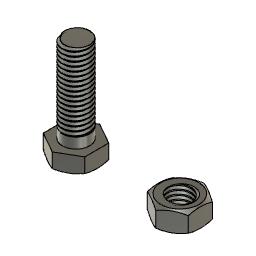
screw v1 (Autodesk Fusion 360 design; units mm, degrees)
Autodesk Fusion 360 part; units mm, degrees
sketch "Sketch1" plane through (0, 0, 0) normal (0, 0, 1) x (1, 0, 0)
  line L0 (6.0104, -3.446) -> (5.9895, 3.4822)
  line L1 (5.9895, 3.4822) -> (-0.0209, 6.9282)
  line L2 (-0.0209, 6.9282) -> (-6.0104, 3.446)
  line L3 (-6.0104, 3.446) -> (-5.9895, -3.4822)
  line L4 (-5.9895, -3.4822) -> (0.0209, -6.9282)
  line L5 (0.0209, -6.9282) -> (6.0104, -3.446)
  circle A0 centre (0, 0) radius 5.5
  circle A1 centre (0, 0) radius 4
  dimension "d1" = 6
  dimension "d2" = 11
  dimension "d3" = 8
  constraint coincident A0.centre A1.centre
  measures "d1" distance of A0.centre L5
  measures "d2" diameter of A0
  measures "d3" diameter of A1
extrude "Extrude1" add sketch "Sketch1" along normal blind 5 contours L0 L1 L2 L3 L4 L5 | A0 | A1 makes body 1
extrude "Extrude2" cut sketch "Sketch1" along normal blind 12.535 draft 60 contours A0 keep common part bodies 1
extrude "Extrude3" add sketch "Sketch1" along normal blind 30 contours A1 bodies 1
thread "Thread1" "ISO Metric profile 8.0 M8x1.25 6g" major diameter 7.866 minor diameter 6.4455 pitch 1.25 angle 60 modelled right hand crest width 0.1833 on face at (3.9801, 0.3983, 13.3333) from (0, 0, 8) to (0, 0, 30) crest through (3.933, 0, 4.6875) on bodies 1
sketch "Sketch2" plane through (0, 0, 0) normal (0, 0, 1) x (1, 0, 0)
  line L0 (35.9472, -3.4041) -> (36.0159, 3.5237)
  line L1 (36.0159, 3.5237) -> (30.0505, 7.0471)
  line L2 (30.0505, 7.0471) -> (24.0164, 3.6427)
  line L3 (24.0164, 3.6427) -> (23.9478, -3.2852)
  line L4 (23.9478, -3.2852) -> (29.9132, -6.8086)
  line L5 (29.9132, -6.8086) -> (35.9472, -3.4041)
  circle A0 centre (29.9818, 0.1193) radius 5.5
  circle A1 centre (29.9818, 0.1193) radius 4
  point P0 (29.9818, 0.1193)
  dimension "d12" = 6
  dimension "d13" = 11
  dimension "d14" = 8
  constraint coincident P0 A0.centre
  constraint concentric A0 A1
  measures "d12" distance of P0 L5
  measures "d13" diameter of A0
  measures "d14" diameter of A1
extrude "Extrude4" add sketch "Sketch2" along normal blind 6 separate body contours L0 L1 L2 L3 L4 L5 | A0 makes body 2
sketch "Sketch3" plane through (0, 0, 0) normal (0, 0, 1) x (1, 0, 0)
  circle A0 centre (29.976, -0.0398) radius 5.5
  dimension "d17" = 11
  measures "d17" diameter of A0
extrude "Extrude5" cut sketch "Sketch3" along normal blind 8.942 draft 60 keep common part bodies 2
sketch "Sketch4" plane through (0, 0, 6) normal (0, 0, 1) x (-1, 0, 0)
  circle A0 centre (-29.9818, -0.1193) radius 4
  line L0 (-29.9132, 6.8086) -> (-35.9472, 3.4041)
  line L1 (-35.9472, 3.4041) -> (-36.0159, -3.5237)
  line L2 (-36.0159, -3.5237) -> (-30.0505, -7.0471)
  line L3 (-30.0505, -7.0471) -> (-24.0164, -3.6427)
  line L4 (-24.0164, -3.6427) -> (-23.9478, 3.2852)
  line L5 (-23.9478, 3.2852) -> (-29.9132, 6.8086)
  circle A1 centre (-29.9818, -0.1193) radius 5.5
  dimension "d20" = 11
  constraint concentric A0 A1
  measures "d20" diameter of A1
extrude "Extrude6" cut sketch "Sketch4" against normal blind 9.465 draft 60 contours A1 keep common part bodies 2
thread "Thread2" "ISO Metric profile 8.0 M8x1.25 6H" major diameter 8.17 minor diameter 6.7795 pitch 1.25 angle 60 modelled right hand crest width 0.343 on face at (33.9619, -0.279, 2) crest through (33.3716, 0.1193, 0.3125) on bodies 2
